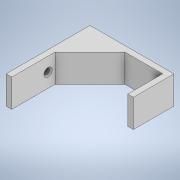
# Autodesk Inventor part: corner
Saved by Autodesk Inventor 2021.1 (Build 251245010, 245A)
## iProperties
Created: 2021-07-16
Part Number: corner
Material: Типовые
Document SubType Name: Modeling
Designer: User
Density: 1 g/cm^3
Appearance: По умолчанию
Author: User
Autodesk Inventor part; units mm, degrees
ref_plane "YZ Plane" through (0, 0, 0) normal (1, 0, 0) x (0, 1, 0)
ref_plane "XZ Plane" through (0, 0, 0) normal (0, 1, 0) x (-1, 0, 0)
ref_plane "XY Plane" through (0, 0, 0) normal (0, 0, 1) x (1, 0, 0)
sketch "Эскиз1" plane through (0, 0, 0) normal (0, 1, 0) x (-1, 0, 0)
  line L0 (0, 0) -> (-4, 0)
  line L1 (-4, 29) -> (-4, 60)
  line L2 (-4, 60) -> (0, 60)
  line L3 (0, 60) -> (0, 0)
  line L4 (0, 0) -> (-60, 0)
  line L5 (-60, 0) -> (-60, 4)
  line L6 (-60, 4) -> (-29, 4)
  line L7 (0, 4) -> (0, 0)
  line L8 (-4, 29) -> (-29, 4)
  dimension "d0" = 4
  dimension "d1" = 60
  dimension "d2" = 60
  dimension "d3" = 4
  dimension "d4" = 25
  dimension "d5" = 25
  constraints: 18 end point, 4 parallel, 2 horizontal, 2 perpendicular
  measures "d0" distance of L1.end L2.end
  measures "d1" distance of L0.end L1.end
  measures "d2" distance of L5.end L7.start
  measures "d3" distance of L4.end L5.end
  measures "d4" distance from line of L1.start L6
  measures "d5" distance from line of L6.end L1
extrude "Выдавливание1" add sketch "Эскиз1" along normal blind 20
sketch "Эскиз2" plane through (4, 0, 60) normal (1, 0, 0) x (0, 0, -1)
  line L0 (0, 20) -> (31, 20) projected
  line L1 (0, 0) -> (0, 20) projected
  circle A0 centre (26, 10) radius 2
  line L2 (31, 0) -> (31, 20) projected
  point P0 (60, 0)
  dimension "d11" = 4
  dimension "d12" = 5
  constraints: 1 centre point
  measures "d11" diameter of A0
  measures "d12" distance from line of L2 A0.centre
extrude "Выдавливание2" cut sketch "Эскиз2" against normal blind 10
chamfer "Фаска1" distance 1 angle 45 1 edges at (4, 10, 36)
sketch "Эскиз3" plane through (29, 0, 4) normal (0, 0, 1) x (1, 0, 0)
  line L0 (31, 0) -> (31, 20) projected
  line L1 (31, 20) -> (27, 20)
  line L2 (27, 20) -> (27, 0)
  line L3 (27, 0) -> (31, 0)
  line L4 (31, 0) -> (31, 20)
  line L5 (0, 0) -> (31, 0) projected
  point P0 (-29, 0)
  point P1 (29, 0)
  dimension "d18" = 4
  constraints: 8 end point, 2 parallel, 1 horizontal, 1 midpoint, 1 perpendicular, 1 point on line
  measures "d18" distance of L3.end L2.end
extrude "Выдавливание3" add sketch "Эскиз3" along normal blind 25
